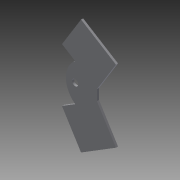
# Autodesk Inventor part: drzak_buzirka
Saved by Autodesk Inventor 2015 (Build 190159000, 159)
## iProperties
Created: 2016-01-15
Part Number: drzak_buzirka
Material: Generic
Document SubType Name: Modeling
Designer: Turboslimak
Density: 1 g/cm^3
Appearance: Default
Author: Turboslimak
Autodesk Inventor part; units mm, degrees
ref_plane "YZ Plane" through (0, 0, 0) normal (1, 0, 0) x (0, 1, 0)
ref_plane "XZ Plane" through (0, 0, 0) normal (0, 1, 0) x (-1, 0, 0)
ref_plane "XY Plane" through (0, 0, 0) normal (0, 0, 1) x (1, 0, 0)
sketch "Sketch1" plane through (0, 0, 0) normal (0, 1, 0) x (-1, 0, 0)
  line L0 (-21, -5) -> (-21, 5)
  line L1 (0, -18) -> (-21, -5)
  line L2 (0, 18) -> (-21, 5)
  line L3 (-21, -5) -> (-39.4224, -34.7593)
  line L4 (0, -18) -> (-18.4224, -47.7593)
  line L5 (-18.4224, -47.7593) -> (-39.4224, -34.7593)
  line L6 (-21, 5) -> (-39.4224, 34.7593)
  line L7 (0, 18) -> (-18.4224, 47.7593)
  line L8 (-18.4224, 47.7593) -> (-39.4224, 34.7593)
  arc A0 (0, -18) -> (0, 18) centre (-13.5, 0) ccw
  circle A1 centre (0, 0) radius 3
  line L9 (-18.4224, -47.7593) -> (0, -18)
  line L10 (0, -18) -> (12.754, -25.8953)
  line L11 (12.754, -25.8953) -> (-5.6684, -55.6546)
  line L12 (-5.6684, -55.6546) -> (-18.4224, -47.7593)
  line L13 (0, 18) -> (-18.4224, 47.7593)
  line L14 (-18.4224, 47.7593) -> (-5.6684, 55.6546)
  line L15 (-5.6684, 55.6546) -> (12.754, 25.8953)
  line L16 (12.754, 25.8953) -> (0, 18)
  point P0 (-21, 0)
  dimension "d5" = 10
  dimension "d6" = 35
  dimension "d7" = 35
  dimension "d8" = 35
  dimension "d9" = 35
  dimension "d10" = 36
  dimension "d12" = 6
  dimension "d13" = 15
  dimension "d14" = 15
  constraints: 34 end point, 6 equal length, 6 perpendicular, 2 centre point, 2 point on circle, 1 midpoint, 1 other
  measures "d5" distance of L0.start L0.end
  measures "d6" distance of L0.start L3.end
  measures "d7" distance of L1.start L4.end
  measures "d8" distance of L2.start L7.end
  measures "d9" distance of L0.end L6.end
  measures "d10" distance of L1.start L2.start
  measures "d12" diameter of A1
  measures "d13" distance of L1.start L10.end
  measures "d14" distance of L7.end L14.end
extrude "Extrusion1" add sketch "Sketch1" along normal blind 2
body "Solid1"
